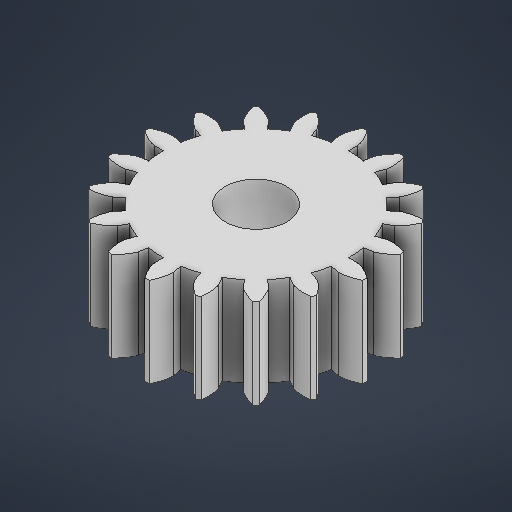
# Autodesk Inventor part: 36mm_18N_Gear
Saved by Autodesk Inventor 2026.2 (Build 302298000, 298)
## iProperties
Created: 2025-12-19
Part Number: 36mm_18N_Gear
Material: Generic
Document SubType Name: Modeling
Designer: Cobble
Density: 1 g/cm^3
Appearance: Default
Author: Cobble
Autodesk Inventor part; units mm, degrees
ref_plane "YZ Plane" through (0, 0, 0) normal (1, 0, 0) x (0, 1, 0)
ref_plane "XZ Plane" through (0, 0, 0) normal (0, 1, 0) x (-1, 0, 0)
ref_plane "XY Plane" through (0, 0, 0) normal (0, 0, 1) x (1, 0, 0)
sketch "Sketch1" plane through (0, 0, 0) normal (0, 0, 1) x (1, 0, 0)
  circle A0 centre (0, 0) radius 18 construction
  circle A1 centre (0, 0) radius 20
  circle A2 centre (0, 0) radius 16.9145 construction
  line L0 (0, 0) -> (0, 20)
  line L1 (0, 0) -> (-6.8404, 18.7939)
  line L2 (0, 0) -> (-12.8558, 15.3209)
  line L3 (0, 0) -> (-17.3205, 10)
  line L4 (0, 0) -> (-19.6962, 3.473)
  line L5 (0, 0) -> (-19.6962, -3.473)
  line L6 (0, 0) -> (-17.3205, -10)
  line L7 (0, 0) -> (-12.8558, -15.3209)
  line L8 (0, 0) -> (-6.8404, -18.7939)
  line L9 (0, 0) -> (0, -20)
  line L10 (0, 0) -> (6.8404, -18.7939)
  line L11 (0, 0) -> (12.8558, -15.3209)
  line L12 (0, 0) -> (17.3205, -10)
  line L13 (0, 0) -> (19.6962, -3.473)
  line L14 (0, 0) -> (19.6962, 3.473)
  line L15 (0, 0) -> (17.3205, 10)
  line L16 (0, 0) -> (12.8558, 15.3209)
  line L17 (0, 0) -> (6.8404, 18.7939)
  line L18 (-5.7851, 15.8944) -> (-0.2372, 17.9137) construction
  line L19 (-10.8724, 12.9573) -> (-1.827, 20.5473) construction
  line L20 (-14.6484, 8.4573) -> (-5.7924, 23.7963) construction
  line L21 (-16.6575, 2.9372) -> (-12.5567, 26.1944) construction
  line L22 (-16.6575, -2.9372) -> (-21.7836, 26.1344) construction
  spline S0 degree 4 poles (0, 16.9145) (0.0276, 17.5554) (-1.8377, 22.4564) (-8.2459, 26.2252) (-16.545, 27.1665) (-21.7836, 26.1344) knots 0 0 0 0 0 0.384317 1 1 1 1 1
  line L23 (0, 0) -> (3.1257, 17.7265)
  line L24 (0, 0) -> (18, 0)
  line L25 (0, 0) -> (-3.1257, 17.7265)
  line L26 (0, 0) -> (-9, 15.5885)
  line L27 (0, 0) -> (-13.7888, 11.5702)
  line L28 (0, 0) -> (-16.9145, 6.1564)
  line L29 (0, 0) -> (-18, 0)
  line L30 (0, 0) -> (-16.9145, -6.1564)
  line L31 (0, 0) -> (-13.7888, -11.5702)
  line L32 (0, 0) -> (-9, -15.5885)
  line L33 (0, 0) -> (-3.1257, -17.7265)
  line L34 (0, 0) -> (3.1257, -17.7265)
  line L35 (0, 0) -> (9, -15.5885)
  line L36 (0, 0) -> (13.7888, -11.5702)
  line L37 (0, 0) -> (16.9145, -6.1564)
  line L38 (0, 0) -> (18, 0)
  line L39 (0, 0) -> (16.9145, 6.1564)
  line L40 (0, 0) -> (13.7888, 11.5702)
  line L41 (0, 0) -> (9, 15.5885)
  line L42 (2.9372, 16.6575) -> (-2.8771, 17.6827) construction
  line L43 (8.4573, 14.6484) -> (-1.7688, 20.5524) construction
  line L44 (12.9573, 10.8724) -> (1.5722, 24.4406) construction
  line L45 (15.8944, 5.7851) -> (7.8173, 27.9769) construction
  line L46 (16.9145, 0) -> (16.9145, 29.52) construction
  spline S1 degree 4 poles (-2.9372, 16.6575) (-3.0757, 17.2839) (-2.0897, 22.4344) (3.5667, 27.2587) (11.5762, 29.6268) (16.9145, 29.52) knots 0 0 0 0 0 0.384317 1 1 1 1 1
  circle A3 centre (0, 0) radius 15.5
  spline S2 degree 4 poles (-5.7851, 15.8944) (-5.9784, 16.5062) (-9.4075, 20.4736) (-16.7182, 21.8234) (-24.8387, 19.8695) (-29.4084, 17.1078) knots 0 0 0 0 0 0.384317 1 1 1 1 1
  spline S3 degree 4 poles (-8.4572, 14.6484) (-8.8016, 15.1897) (-9.6367, 20.3667) (-5.9714, 26.8347) (0.7451, 31.7994) (5.798, 33.5248) knots 0 0 0 0 0 0.384317 1 1 1 1 1
  spline S4 degree 4 poles (-10.8724, 12.9573) (-11.2633, 13.466) (-15.8425, 16.0214) (-23.174, 14.7893) (-30.1365, 10.1759) (-33.4861, 6.0178) knots 0 0 0 0 0 0.384317 1 1 1 1 1
  spline S5 degree 4 poles (-12.9573, 10.8724) (-13.466, 11.2633) (-16.0214, 15.8425) (-14.7893, 23.174) (-10.1759, 30.1365) (-6.0178, 33.4861) knots 0 0 0 0 0 0.384317 1 1 1 1 1
  spline S6 degree 4 poles (-14.6484, 8.4573) (-15.1897, 8.8016) (-20.3667, 9.6367) (-26.8347, 5.9714) (-31.7994, -0.7451) (-33.5248, -5.798) knots 0 0 0 0 0 0.384317 1 1 1 1 1
  spline S7 degree 4 poles (-15.8944, 5.7851) (-16.5062, 5.9784) (-20.4736, 9.4075) (-21.8234, 16.7182) (-19.8695, 24.8387) (-17.1078, 29.4084) knots 0 0 0 0 0 0.384317 1 1 1 1 1
  spline S8 degree 4 poles (-16.6575, 2.9372) (-17.2839, 3.0757) (-22.4344, 2.0897) (-27.2587, -3.5667) (-29.6268, -11.5762) (-29.52, -16.9145) knots 0 0 0 0 0 0.384317 1 1 1 1 1
  spline S9 degree 4 poles (-16.9145, 0) (-17.5554, -0.0276) (-22.4564, 1.8377) (-26.2252, 8.2459) (-27.1665, 16.545) (-26.1344, 21.7836) knots 0 0 0 0 0 0.384317 1 1 1 1 1
  spline S10 degree 4 poles (-16.6575, -2.9372) (-17.2935, -3.0213) (-21.7962, -5.7093) (-24.3949, -12.6746) (-23.8808, -21.011) (-21.9546, -25.9909) knots 0 0 0 0 0 0.384317 1 1 1 1 1
  spline S11 degree 4 poles (-15.8944, -5.7851) (-16.4873, -6.0303) (-21.7307, -5.9536) (-27.464, -1.2209) (-31.1869, 6.2557) (-32.0087, 11.5314) knots 0 0 0 0 0 0.384317 1 1 1 1 1
  spline S12 degree 4 poles (-14.6484, -8.4572) (-15.2173, -8.7538) (-18.529, -12.8198) (-18.5888, -20.2538) (-15.2544, -27.9116) (-11.7412, -31.9323) knots 0 0 0 0 0 0.384317 1 1 1 1 1
  spline S13 degree 4 poles (-12.9573, -10.8724) (-13.4305, -11.3056) (-18.3839, -13.0269) (-25.3901, -10.5405) (-31.4456, -4.7881) (-34.0223, -0.1116) knots 0 0 0 0 0 0.384317 1 1 1 1 1
  spline S14 degree 4 poles (-10.8724, -12.9573) (-11.3056, -13.4305) (-13.0269, -18.3839) (-10.5405, -25.3901) (-4.7881, -31.4456) (-0.1116, -34.0223) knots 0 0 0 0 0 0.384317 1 1 1 1 1
  spline S15 degree 4 poles (-8.4573, -14.6484) (-8.7538, -15.2173) (-12.8198, -18.529) (-20.2538, -18.5888) (-27.9116, -15.2544) (-31.9323, -11.7412) knots 0 0 0 0 0 0.384317 1 1 1 1 1
  spline S16 degree 4 poles (-5.7851, -15.8944) (-6.0303, -16.4873) (-5.9536, -21.7307) (-1.2209, -27.464) (6.2557, -31.1869) (11.5314, -32.0087) knots 0 0 0 0 0 0.384317 1 1 1 1 1
  spline S17 degree 4 poles (-2.9372, -16.6575) (-3.0213, -17.2935) (-5.7093, -21.7962) (-12.6746, -24.3949) (-21.011, -23.8808) (-25.9909, -21.9546) knots 0 0 0 0 0 0.384317 1 1 1 1 1
  spline S18 degree 4 poles (0, -16.9145) (-0.0276, -17.5554) (1.8377, -22.4564) (8.2459, -26.2252) (16.545, -27.1665) (21.7836, -26.1344) knots 0 0 0 0 0 0.384317 1 1 1 1 1
  spline S19 degree 4 poles (2.9372, -16.6575) (3.0757, -17.2839) (2.0897, -22.4344) (-3.5667, -27.2587) (-11.5762, -29.6268) (-16.9145, -29.52) knots 0 0 0 0 0 0.384317 1 1 1 1 1
  spline S20 degree 4 poles (5.7851, -15.8944) (5.9784, -16.5062) (9.4075, -20.4736) (16.7182, -21.8234) (24.8387, -19.8695) (29.4084, -17.1078) knots 0 0 0 0 0 0.384317 1 1 1 1 1
  spline S21 degree 4 poles (8.4572, -14.6484) (8.8016, -15.1897) (9.6367, -20.3667) (5.9714, -26.8347) (-0.7451, -31.7994) (-5.798, -33.5248) knots 0 0 0 0 0 0.384317 1 1 1 1 1
  spline S22 degree 4 poles (10.8724, -12.9573) (11.2633, -13.466) (15.8425, -16.0214) (23.174, -14.7893) (30.1365, -10.1759) (33.4861, -6.0178) knots 0 0 0 0 0 0.384317 1 1 1 1 1
  spline S23 degree 4 poles (12.9573, -10.8724) (13.466, -11.2633) (16.0214, -15.8425) (14.7893, -23.174) (10.1759, -30.1365) (6.0178, -33.4861) knots 0 0 0 0 0 0.384317 1 1 1 1 1
  spline S24 degree 4 poles (14.6484, -8.4573) (15.1897, -8.8016) (20.3667, -9.6367) (26.8347, -5.9714) (31.7994, 0.7451) (33.5248, 5.798) knots 0 0 0 0 0 0.384317 1 1 1 1 1
  spline S25 degree 4 poles (15.8944, -5.7851) (16.5062, -5.9784) (20.4736, -9.4075) (21.8234, -16.7182) (19.8695, -24.8387) (17.1078, -29.4084) knots 0 0 0 0 0 0.384317 1 1 1 1 1
  spline S26 degree 4 poles (16.6575, -2.9372) (17.2839, -3.0757) (22.4344, -2.0897) (27.2587, 3.5667) (29.6268, 11.5762) (29.52, 16.9145) knots 0 0 0 0 0 0.384317 1 1 1 1 1
  spline S27 degree 4 poles (16.9145, 0) (17.5554, 0.0276) (22.4564, -1.8377) (26.2252, -8.2459) (27.1665, -16.545) (26.1344, -21.7836) knots 0 0 0 0 0 0.384317 1 1 1 1 1
  spline S28 degree 4 poles (16.6575, 2.9372) (17.2935, 3.0213) (21.7962, 5.7093) (24.3949, 12.6746) (23.8808, 21.011) (21.9546, 25.9909) knots 0 0 0 0 0 0.384317 1 1 1 1 1
  spline S29 degree 4 poles (15.8944, 5.7851) (16.4873, 6.0303) (21.7307, 5.9536) (27.464, 1.2209) (31.1869, -6.2557) (32.0087, -11.5314) knots 0 0 0 0 0 0.384317 1 1 1 1 1
  spline S30 degree 4 poles (14.6484, 8.4573) (15.2173, 8.7538) (18.529, 12.8198) (18.5888, 20.2538) (15.2544, 27.9116) (11.7412, 31.9323) knots 0 0 0 0 0 0.384317 1 1 1 1 1
  spline S31 degree 4 poles (12.9573, 10.8724) (13.4305, 11.3056) (18.3839, 13.0269) (25.3901, 10.5405) (31.4456, 4.7881) (34.0223, 0.1116) knots 0 0 0 0 0 0.384317 1 1 1 1 1
  spline S32 degree 4 poles (10.8724, 12.9573) (11.3056, 13.4305) (13.0269, 18.3839) (10.5405, 25.3901) (4.7881, 31.4456) (0.1116, 34.0223) knots 0 0 0 0 0 0.384317 1 1 1 1 1
  spline S33 degree 4 poles (8.4573, 14.6484) (8.7538, 15.2173) (12.8198, 18.529) (20.2538, 18.5888) (27.9116, 15.2544) (31.9323, 11.7412) knots 0 0 0 0 0 0.384317 1 1 1 1 1
  spline S34 degree 4 poles (5.7851, 15.8944) (6.0303, 16.4873) (5.9536, 21.7307) (1.2209, 27.464) (-6.2557, 31.1869) (-11.5314, 32.0087) knots 0 0 0 0 0 0.384317 1 1 1 1 1
  spline S35 degree 4 poles (2.9372, 16.6575) (3.0213, 17.2935) (5.7093, 21.7962) (12.6746, 24.3949) (21.011, 23.8808) (25.9909, 21.9546) knots 0 0 0 0 0 0.384317 1 1 1 1 1
  point P0 (-6.3497, 16.7523)
  point P1 (-8.7444, 18.6833)
  point P2 (-13.5819, 20.3801)
  point P3 (-20.7584, 20.32)
  point P4 (-8.7515, 15.6323)
  point P5 (-8.6914, 18.708)
  point P6 (-6.8818, 23.5044)
  point P7 (-2.2228, 28.9633)
  point P8 (-11.6964, 13.5703)
  point P9 (-14.6071, 14.5658)
  point P10 (-19.7332, 14.5057)
  point P11 (-26.4564, 11.9948)
  point P12 (-13.5703, 11.6964)
  point P13 (-14.5658, 14.6071)
  point P14 (-14.5057, 19.7332)
  point P15 (-11.9948, 26.4564)
  point P16 (-15.6323, 8.7515)
  point P17 (-18.708, 8.6914)
  point P18 (-23.5044, 6.8818)
  point P19 (-28.9633, 2.2228)
  point P20 (-16.7523, 6.3497)
  point P21 (-18.6833, 8.7444)
  point P22 (-20.3801, 13.5819)
  point P23 (-20.32, 20.7584)
  point P24 (-17.6827, 2.8771)
  point P25 (-20.5524, 1.7688)
  point P26 (-24.4406, -1.5722)
  point P27 (-27.9769, -7.8173)
  point P28 (-17.9137, 0.2372)
  point P29 (-20.5473, 1.827)
  point P30 (-23.7963, 5.7924)
  point P31 (-26.1944, 12.5567)
  point P32 (-17.6004, -3.3442)
  point P33 (-19.9179, -5.3672)
  point P34 (-22.4289, -9.8366)
  point P35 (-23.616, -16.9145)
  point P36 (-16.9145, -5.904)
  point P37 (-19.933, -5.3108)
  point P38 (-24.3423, -2.6957)
  point P39 (-28.9093, 2.8404)
  point P40 (-15.3952, -9.1622)
  point P41 (-16.881, -11.8559)
  point P42 (-17.712, -16.9145)
  point P43 (-16.4067, -23.9716)
  point P44 (-13.8751, -11.333)
  point P45 (-16.9145, -11.808)
  point P46 (-21.9523, -10.8587)
  point P47 (-28.1373, -7.2185)
  point P48 (-11.333, -13.8751)
  point P49 (-11.808, -16.9145)
  point P50 (-10.8587, -21.9523)
  point P51 (-7.2185, -28.1373)
  point P52 (-9.1622, -15.3952)
  point P53 (-11.8559, -16.881)
  point P54 (-16.9145, -17.712)
  point P55 (-23.9716, -16.4067)
  point P56 (-5.904, -16.9145)
  point P57 (-5.3108, -19.933)
  point P58 (-2.6957, -24.3423)
  point P59 (2.8404, -28.9093)
  point P60 (-3.3442, -17.6004)
  point P61 (-5.3672, -19.9179)
  point P62 (-9.8366, -22.4289)
  point P63 (-16.9145, -23.616)
  point P64 (0.2372, -17.9137)
  point P65 (1.827, -20.5473)
  point P66 (5.7924, -23.7963)
  point P67 (12.5567, -26.1944)
  point P68 (2.8771, -17.6827)
  point P69 (1.7688, -20.5524)
  point P70 (-1.5722, -24.4406)
  point P71 (-7.8173, -27.9769)
  point P72 (6.3497, -16.7523)
  point P73 (8.7444, -18.6833)
  point P74 (13.5819, -20.3801)
  point P75 (20.7584, -20.32)
  point P76 (8.7515, -15.6323)
  point P77 (8.6914, -18.708)
  point P78 (6.8818, -23.5044)
  point P79 (2.2228, -28.9633)
  point P80 (11.6964, -13.5703)
  point P81 (14.6071, -14.5658)
  point P82 (19.7332, -14.5057)
  point P83 (26.4564, -11.9948)
  point P84 (13.5703, -11.6964)
  point P85 (14.5658, -14.6071)
  point P86 (14.5057, -19.7332)
  point P87 (11.9948, -26.4564)
  point P88 (15.6323, -8.7515)
  point P89 (18.708, -8.6914)
  point P90 (23.5044, -6.8818)
  point P91 (28.9633, -2.2228)
  point P92 (16.7523, -6.3497)
  point P93 (18.6833, -8.7444)
  point P94 (20.3801, -13.5819)
  point P95 (20.32, -20.7584)
  point P96 (17.6827, -2.8771)
  point P97 (20.5524, -1.7688)
  point P98 (24.4406, 1.5722)
  point P99 (27.9769, 7.8173)
  point P100 (17.9137, -0.2372)
  point P101 (20.5473, -1.827)
  point P102 (23.7963, -5.7924)
  point P103 (26.1944, -12.5567)
  point P104 (17.6004, 3.3442)
  point P105 (19.9179, 5.3672)
  point P106 (22.4289, 9.8366)
  point P107 (23.616, 16.9145)
  point P108 (16.9145, 5.904)
  point P109 (19.933, 5.3108)
  point P110 (24.3423, 2.6957)
  point P111 (28.9093, -2.8404)
  point P112 (15.3952, 9.1622)
  point P113 (16.881, 11.8559)
  point P114 (17.712, 16.9145)
  point P115 (16.4067, 23.9716)
  point P116 (13.8751, 11.333)
  point P117 (16.9145, 11.808)
  point P118 (21.9523, 10.8587)
  point P119 (28.1373, 7.2185)
  point P120 (11.333, 13.8751)
  point P121 (11.808, 16.9145)
  point P122 (10.8587, 21.9523)
  point P123 (7.2185, 28.1373)
  point P124 (9.1622, 15.3952)
  point P125 (11.8559, 16.881)
  point P126 (16.9145, 17.712)
  point P127 (23.9716, 16.4067)
  point P128 (5.904, 16.9145)
  point P129 (5.3108, 19.933)
  point P130 (2.6957, 24.3423)
  point P131 (-2.8404, 28.9093)
  point P132 (3.3442, 17.6004)
  point P133 (5.3672, 19.9179)
  point P134 (9.8366, 22.4289)
  point P135 (16.9145, 23.616)
  point P136 (-7.75, 13.4234)
  point P137 (-9.9632, 11.8737)
  point P138 (-10.9161, 13.0093)
  point P139 (-13.8744, 14.4049)
  point P140 (-14.4049, 13.8744)
  point P141 (-13.0093, 10.9161)
  point P142 (-11.8737, 9.9632)
  point P143 (-13.4234, 7.75)
  point P144 (-14.7072, 8.4912)
  point P145 (-17.9644, 8.7909)
  point P146 (-18.2815, 8.1109)
  point P147 (-15.9583, 5.8083)
  point P148 (-14.5652, 5.3013)
  point P149 (-15.2645, 2.6915)
  point P150 (-16.7245, 2.949)
  point P151 (-19.8877, 2.1165)
  point P152 (-19.9531, 1.3691)
  point P153 (-16.9825, 0)
  point P154 (-15.5, 0)
  point P155 (-15.2645, -2.6915)
  point P156 (-16.7245, -2.949)
  point P157 (-19.4122, -4.8131)
  point P158 (-19.218, -5.5378)
  point P159 (-15.9583, -5.8083)
  point P160 (-14.5652, -5.3013)
  point P161 (-13.4234, -7.75)
  point P162 (-14.7072, -8.4912)
  point P163 (-16.5953, -11.1622)
  point P164 (-16.165, -11.7768)
  point P165 (-13.0093, -10.9161)
  point P166 (-11.8737, -9.9632)
  point P167 (-9.9632, -11.8737)
  point P168 (-10.9161, -13.0093)
  point P169 (-11.7768, -16.165)
  point P170 (-11.1622, -16.5953)
  point P171 (-8.4912, -14.7072)
  point P172 (-7.75, -13.4234)
  point P173 (-5.3013, -14.5652)
  point P174 (-5.8083, -15.9583)
  point P175 (-5.5378, -19.218)
  point P176 (-4.8131, -19.4122)
  point P177 (-2.949, -16.7245)
  point P178 (-2.6915, -15.2645)
  point P179 (0, -15.5)
  point P180 (0, -16.9825)
  point P181 (1.3691, -19.9531)
  point P182 (2.1165, -19.8877)
  point P183 (2.949, -16.7245)
  point P184 (2.6915, -15.2645)
  point P185 (5.3013, -14.5652)
  point P186 (5.8083, -15.9583)
  point P187 (8.1109, -18.2815)
  point P188 (8.7909, -17.9644)
  point P189 (8.4912, -14.7072)
  point P190 (7.75, -13.4234)
  point P191 (9.9632, -11.8737)
  point P192 (10.9161, -13.0093)
  point P193 (13.8744, -14.4049)
  point P194 (14.4049, -13.8744)
  point P195 (13.0093, -10.9161)
  point P196 (11.8737, -9.9632)
  point P197 (13.4234, -7.75)
  point P198 (14.7072, -8.4912)
  point P199 (17.9644, -8.7909)
  dimension "d0" = 36
  dimension "d1" = 40
  dimension "d2" = 33.829
  dimension "d22" = 31
  dimension "d5" = 360
  dimension "d7" = 5.904
  dimension "d8" = 11.808
  dimension "d9" = 17.712
  dimension "d10" = 23.616
  dimension "d11" = 29.52
  dimension "d12" = 80
  dimension "d15" = 360
  dimension "d17" = 5.904
  dimension "d18" = 11.808
  dimension "d19" = 17.712
  dimension "d20" = 23.616
  dimension "d21" = 29.52
  dimension "d25" = 360
  constraints: 94 end point, 12 point on line, 10 perpendicular, 6 coincident, 2 vertical, 1 equal length, 1 horizontal, 626 other
  measures "d7" distance of L18.start L18.end
  measures "d8" distance of L19.start L19.end
  measures "d9" distance of L20.start L20.end
  measures "d10" distance of L21.start L21.end
  measures "d11" distance of L22.start L22.end
  measures "d12" angle of L24 L23
  measures "d17" distance of L42.start L42.end
  measures "d18" distance of L43.start L43.end
  measures "d19" distance of L44.start L44.end
  measures "d20" distance of L45.start L45.end
  measures "d21" distance of L46.start L46.end
extrude "Extrusion1" add sketch "Sketch1" along normal blind 15 contours L14 A3 L39 S29 A1 S28 | A1 S26 L13 A3 L24 S27 | A3 L24 L14 | L14 L39 A3 | A3 L13 L24 | L25 A3 L0 | L26 A3 L1 | L27 A3 L2 | L28 A3 L3 | L29 A3 L4 | L30 A3 L5 | L31 A3 L6 | L32 A3 L7 | L33 A3 L8 | L34 A3 L9 | L35 A3 L10 | L36 A3 L11 | L37 A3 L12 | L40 A3 L15 | L41 A3 L16 | L23 A3 L17 | L0 A3 L23 | L1 A3 L25 | L2 A3 L26 | L3 A3 L27 | L4 A3 L28 | L5 A3 L29 | L6 A3 L30 | L7 A3 L31 | L8 A3 L32 | L9 A3 L33 | L10 A3 L34 | L11 A3 L35 | L12 A3 L36 | L13 A3 L37 | L15 A3 L39 | L16 A3 L40 | L17 A3 L41 | A1 S24 L12 A3 L37 S25 | S30 L15 A3 L40 S31 A1 | A3 L25 S1 A1 S0 L0 | A3 L26 S3 A1 S2 L1 | A3 L27 S5 A1 S4 L2 | A3 L28 S7 A1 S6 L3 | A3 L29 S9 A1 S8 L4 | A3 L30 S11 A1 S10 L5 | A3 L31 S13 A1 S12 L6 | A3 L32 S15 A1 S14 L7 | A3 L33 S17 A1 S16 L8 | A3 L34 S19 A1 S18 L9 | A3 L35 S21 A1 S20 L10 | A3 L36 S23 A1 S22 L11 | A3 L41 S33 A1 S32 L16 | A3 L23 S35 A1 S34 L17
sketch "Sketch2" plane through (0, 0, 15) normal (0, 0, 1) x (1, 0, 0)
  circle A0 centre (0, 0) radius 5.15
  dimension "d29" = 10.3
  constraints: 1 centre point, 1 coincident
  measures "d29" diameter of A0
extrude "Extrusion2" cut sketch "Sketch2" against normal through all
equation "\"d8\" = 2 * d7"
equation "\"d9\" = 3 * d7"
equation "\"d10\" = 2 * d8"
equation "\"d11\" = 5 * d7"
equation "\"d17\" = d7"
equation "\"d18\" = d8"
equation "\"d19\" = d9"
equation "\"d20\" = d10"
equation "\"d21\" = d11"
body "Solid1"
